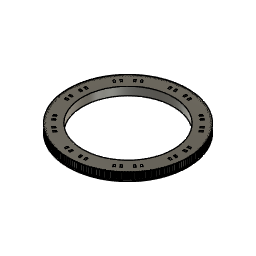
180 tooth pulley v3 (Autodesk Fusion 360 design; units mm, degrees)
Autodesk Fusion 360 part; units mm, degrees
(part 1 of 6)
sketch "Sketch1" plane through (0, 0, 0) normal (0, 0, 1) x (1, 0, 0)
  circle A0 centre (0, 0) radius 140.9967 construction
  circle A1 centre (0, 0) radius 143.2467 construction
  line L0 (0, 0) -> (143.2467, 0) construction
  line L1 (0, 0) -> (143.2249, 2.5) construction
  line L2 (143.2467, 0) -> (143.2467, 0.325)
  arc A2 (143.2467, 0.325) -> (142.786, 0.8235) centre (142.7467, 0.325) ccw
  arc A3 (140.9752, 2.4607) -> (142.786, 0.8235) centre (142.9432, 2.8173) ccw
  arc A4 (142.786, -0.8235) -> (140.9752, -2.4607) centre (142.9432, -2.8173) ccw
  arc A5 (142.786, -0.8235) -> (143.2467, -0.325) centre (142.7467, -0.325) ccw
  line L3 (143.2467, 0) -> (143.2467, -0.325)
  arc A6 (140.8035, 7.3792) -> (142.6703, 5.8061) centre (142.7578, 7.8042) ccw
  arc A7 (143.1481, 5.324) -> (142.6703, 5.8061) centre (142.6484, 5.3066) ccw
  line L4 (143.1595, 4.9992) -> (143.1481, 5.324)
  line L5 (143.1595, 4.9992) -> (143.1708, 4.6744)
  arc A8 (142.7278, 4.1602) -> (143.1708, 4.6744) centre (142.6711, 4.657) ccw
  arc A9 (142.7278, 4.1602) -> (140.9752, 2.4607) centre (142.9545, 2.1731) ccw
  arc A10 (140.4602, 12.2887) -> (142.3808, 10.7817) centre (142.3985, 12.7816) ccw
  arc A11 (142.8751, 10.3166) -> (142.3808, 10.7817) centre (142.3763, 10.2817) ccw
  line L6 (142.8978, 9.9924) -> (142.8751, 10.3166)
  line L7 (142.8978, 9.9924) -> (142.9205, 9.6682)
  arc A12 (142.4956, 9.1388) -> (142.9205, 9.6682) centre (142.4217, 9.6333) ccw
  arc A13 (142.4956, 9.1388) -> (140.8035, 7.3792) centre (142.7915, 7.1608) ccw
  arc A14 (139.9458, 17.1832) -> (141.9177, 15.7441) centre (141.8657, 17.7435) ccw
  arc A15 (142.428, 15.2966) -> (141.9177, 15.7441) centre (141.9308, 15.2443) ccw
  line L8 (142.462, 14.9734) -> (142.428, 15.2966)
  line L9 (142.462, 14.9734) -> (142.496, 14.6501)
  arc A16 (142.0899, 14.1063) -> (142.496, 14.6501) centre (141.9987, 14.5979) ccw
  arc A17 (142.0899, 14.1063) -> (140.4602, 12.2887) centre (142.4546, 12.1398) ccw
  arc A18 (139.2608, 22.0567) -> (141.2818, 20.6874) centre (141.16, 22.6837) ccw
  arc A19 (141.8074, 20.2579) -> (141.2818, 20.6874) centre (141.3123, 20.1883) ccw
  line L10 (141.8527, 19.9361) -> (141.8074, 20.2579)
  line L11 (141.8527, 19.9361) -> (141.8979, 19.6143)
  arc A20 (141.511, 19.0565) -> (141.8979, 19.6143) centre (141.4028, 19.5447) ccw
  arc A21 (141.511, 19.0565) -> (139.9458, 17.1832) centre (141.9442, 17.104) ccw
  arc A22 (138.4062, 26.9034) -> (140.4738, 25.6055) centre (140.2824, 27.5963) ccw
  arc A23 (141.014, 25.1946) -> (140.4738, 25.6055) centre (140.5216, 25.1078) ccw
  line L12 (141.0705, 24.8745) -> (141.014, 25.1946)
  line L13 (141.0705, 24.8745) -> (141.1269, 24.5545)
  arc A24 (140.7598, 23.9836) -> (141.1269, 24.5545) centre (140.6345, 24.4676) ccw
  arc A25 (140.7598, 23.9836) -> (139.2608, 22.0567) centre (141.2608, 22.0474) ccw
  arc A26 (137.383, 31.7174) -> (139.4946, 30.4923) centre (139.2338, 32.4753) ccw
  arc A27 (140.0489, 30.1006) -> (139.4946, 30.4923) centre (139.5598, 29.9966) ccw
  line L14 (140.1164, 29.7827) -> (140.0489, 30.1006)
  line L15 (140.1164, 29.7827) -> (140.184, 29.4648)
  arc A28 (139.837, 28.8814) -> (140.184, 29.4648) centre (139.6949, 29.3608) ccw
  arc A29 (139.837, 28.8814) -> (138.4062, 26.9034) centre (140.4053, 26.9639) ccw
  arc A30 (136.1924, 36.4926) -> (138.3455, 35.3421) centre (138.0156, 37.3147) ccw
  arc A31 (138.9131, 34.9699) -> (138.3455, 35.3421) centre (138.4279, 34.8489) ccw
  line L16 (138.9917, 34.6545) -> (138.9131, 34.9699)
  line L17 (138.9917, 34.6545) -> (139.0703, 34.3392)
  arc A32 (138.7439, 33.7441) -> (139.0703, 34.3392) centre (138.5852, 34.2182) ccw
  arc A33 (138.7439, 33.7441) -> (137.383, 31.7174) centre (139.3787, 31.8475) ccw
  arc A34 (134.8358, 41.2235) -> (137.0278, 40.1487) centre (136.6293, 42.1086) ccw
  arc A35 (137.608, 39.7966) -> (137.0278, 40.1487) centre (137.1274, 39.6587) ccw
  line L18 (137.6976, 39.4841) -> (137.608, 39.7966)
  line L19 (137.6976, 39.4841) -> (137.7872, 39.1717)
  arc A36 (137.4817, 38.5656) -> (137.7872, 39.1717) centre (137.3065, 39.0339) ccw
  arc A37 (137.4817, 38.5656) -> (136.1924, 36.4926) centre (138.1824, 36.6924) ccw
  arc A38 (133.315, 45.904) -> (135.5431, 44.9065) centre (135.0765, 46.8513) ccw
  arc A39 (136.1353, 44.5748) -> (135.5431, 44.9065) centre (135.6598, 44.4203) ccw
  line L20 (136.2357, 44.2657) -> (136.1353, 44.5748)
  line L21 (136.2357, 44.2657) -> (136.3362, 43.9566)
  arc A40 (136.052, 43.3402) -> (136.3362, 43.9566) centre (135.8606, 43.8021) ccw
  arc A41 (136.052, 43.3402) -> (134.8358, 41.2235) centre (136.8177, 41.4925) ccw
  arc A42 (131.6318, 50.5287) -> (133.8933, 49.6095) centre (133.3591, 51.5368) ccw
  arc A43 (134.4967, 49.2987) -> (133.8933, 49.6095) centre (134.0269, 49.1277) ccw
  line L22 (134.6079, 48.9933) -> (134.4967, 49.2987)
  line L23 (134.6079, 48.9933) -> (134.719, 48.6879)
  arc A44 (134.4566, 48.0619) -> (134.719, 48.6879) centre (134.2492, 48.5169) ccw
  arc A45 (134.4566, 48.0619) -> (133.315, 45.904) centre (135.2862, 46.2421) ccw
  arc A46 (129.7882, 55.0918) -> (132.0804, 54.2521) centre (131.4793, 56.1596) ccw
  arc A47 (132.6943, 53.9625) -> (132.0804, 54.2521) centre (132.2307, 53.7752) ccw
  line L24 (132.816, 53.6612) -> (132.6943, 53.9625)
  line L25 (132.816, 53.6612) -> (132.9378, 53.3598)
  arc A48 (132.6974, 52.7251) -> (132.9378, 53.3598) centre (132.4742, 53.1725) ccw
  arc A49 (132.6974, 52.7251) -> (131.6318, 50.5287) centre (133.59, 50.9353) ccw
  arc A50 (127.7864, 59.5878) -> (130.1066, 58.8286) centre (129.4392, 60.7139) ccw
  arc A51 (130.7302, 58.5606) -> (130.1066, 58.8286) centre (130.2734, 58.3572) ccw
  line L26 (130.8624, 58.2637) -> (130.7302, 58.5606)
  line L27 (130.8624, 58.2637) -> (130.9946, 57.9668)
  arc A52 (130.7764, 57.324) -> (130.9946, 57.9668) centre (130.5378, 57.7634) ccw
  arc A53 (130.7764, 57.324) -> (129.7882, 55.0918) centre (131.731, 55.5665) ccw
  arc A54 (125.629, 64.0112) -> (127.9742, 63.3334) centre (127.2415, 65.1943) ccw
  arc A55 (128.6068, 63.0873) -> (127.9742, 63.3334) centre (128.1574, 62.8682) ccw
  line L28 (128.7493, 62.7952) -> (128.6068, 63.0873)
  line L29 (128.7493, 62.7952) -> (128.8918, 62.5031)
  arc A56 (128.6962, 61.8532) -> (128.8918, 62.5031) centre (128.4424, 62.2839) ccw
  arc A57 (128.6962, 61.8532) -> (127.7864, 59.5878) centre (129.7115, 60.13) ccw
  arc A58 (123.3185, 68.3566) -> (125.686, 67.761) centre (124.8887, 69.5953) ccw
  arc A59 (126.3268, 67.5372) -> (125.686, 67.761) centre (125.8853, 67.3025) ccw
  line L30 (126.4793, 67.2503) -> (126.3268, 67.5372)
  line L31 (126.4793, 67.2503) -> (126.6319, 66.9633)
  arc A60 (126.4592, 66.3069) -> (126.6319, 66.9633) centre (126.1905, 66.7286) ccw
  arc A61 (126.4592, 66.3069) -> (125.629, 64.0112) centre (127.534, 64.6203) ccw
  arc A62 (120.8578, 72.6187) -> (123.2446, 72.1061) centre (122.3838, 73.9114) ccw
  arc A63 (123.8928, 71.9048) -> (123.2446, 72.1061) centre (123.4598, 71.6548) ccw
  line L32 (124.0553, 71.6234) -> (123.8928, 71.9048)
  line L33 (124.0553, 71.6234) -> (124.2178, 71.3419)
  arc A64 (124.068, 70.6799) -> (124.2178, 71.3419) centre (123.7848, 71.0919) ccw
  arc A65 (124.068, 70.6799) -> (123.3185, 68.3566) centre (125.2011, 69.0318) ccw
  arc A66 (118.2498, 76.7923) -> (120.653, 76.3634) centre (119.7298, 78.1375) ccw
  arc A67 (121.3079, 76.1848) -> (120.653, 76.3634) centre (120.8839, 75.9199) ccw
  line L34 (121.4801, 75.9092) -> (121.3079, 76.1848)
  line L35 (121.4801, 75.9092) -> (121.6523, 75.6336)
  arc A68 (121.5258, 74.9667) -> (121.6523, 75.6336) centre (121.2283, 75.3686) ccw
  arc A69 (121.5258, 74.9667) -> (120.8578, 72.6187) centre (122.7156, 73.3592) ccw
  arc A70 (115.4978, 80.8724) -> (117.9145, 80.5276) centre (116.9299, 82.2684) ccw
  arc A71 (118.5752, 80.372) -> (117.9145, 80.5276) centre (118.1607, 80.0924) ccw
  line L36 (118.7569, 80.1025) -> (118.5752, 80.372)
  line L37 (118.7569, 80.1025) -> (118.9387, 79.8331)
  arc A72 (118.8354, 79.1623) -> (118.9387, 79.8331) centre (118.5241, 79.5535) ccw
  arc A73 (118.8354, 79.1623) -> (118.2498, 76.7923) centre (120.0807, 77.5972) ccw
  arc A74 (112.605, 84.8539) -> (115.0323, 84.5937) centre (113.9875, 86.2991) ccw
  arc A75 (115.698, 84.4612) -> (115.0323, 84.5937) centre (115.2935, 84.1673) ccw
  line L38 (115.889, 84.1983) -> (115.698, 84.4612)
  line L39 (115.889, 84.1983) -> (116.0801, 83.9354)
  arc A76 (116.0003, 83.2613) -> (116.0801, 83.9354) centre (115.6756, 83.6415) ccw
  arc A77 (116.0003, 83.2613) -> (115.4978, 80.8724) centre (117.2994, 81.7407) ccw
  arc A78 (109.575, 88.7321) -> (112.01, 88.5567) centre (110.9063, 90.2247) ccw
  arc A79 (112.6799, 88.4476) -> (112.01, 88.5567) centre (112.2859, 88.1398) ccw
  line L40 (112.88, 88.1915) -> (112.6799, 88.4476)
  line L41 (112.88, 88.1915) -> (113.08, 87.9354)
  arc A80 (113.0239, 87.259) -> (113.08, 87.9354) centre (112.686, 87.6276) ccw
  arc A81 (113.0239, 87.259) -> (112.605, 84.8539) centre (114.3753, 85.7846) ccw
  arc A82 (106.4116, 92.5022) -> (108.8511, 92.4119) centre (107.6899, 94.0403) ccw
  arc A83 (109.5244, 92.3262) -> (108.8511, 92.4119) centre (109.1414, 92.0048) ccw
  line L42 (109.7334, 92.0772) -> (109.5244, 92.3262)
  line L43 (109.7334, 92.0772) -> (109.9423, 91.8283)
  arc A84 (109.9097, 91.1503) -> (109.9423, 91.8283) centre (109.5592, 91.5069) ccw
  arc A85 (109.9097, 91.1503) -> (109.575, 88.7321) centre (111.3118, 89.724) ccw
  arc A86 (103.1185, 96.1595) -> (105.5597, 96.1544) centre (104.3424, 97.7413) ccw
  arc A87 (106.2356, 96.0923) -> (105.5597, 96.1544) centre (105.864, 95.7577) ccw
  line L44 (106.4531, 95.8508) -> (106.2356, 96.0923)
  line L45 (106.4531, 95.8508) -> (106.6705, 95.6092)
  arc A88 (106.6617, 94.9306) -> (106.6705, 95.6092) centre (106.299, 95.2747) ccw
  arc A89 (106.6617, 94.9306) -> (106.4116, 92.5022) centre (108.1126, 93.554) ccw
  arc A90 (99.6997, 99.6997) -> (102.1396, 99.7798) centre (100.8677, 101.3233) ccw
  arc A91 (102.8173, 99.7413) -> (102.1396, 99.7798) centre (102.4576, 99.394) ccw
  line L46 (103.0431, 99.5075) -> (102.8173, 99.7413)
  line L47 (103.0431, 99.5075) -> (103.2688, 99.2737)
  arc A92 (103.2837, 98.5952) -> (103.2688, 99.2737) centre (102.9092, 98.9264) ccw
  arc A93 (103.2837, 98.5952) -> (103.1185, 96.1595) centre (104.7818, 97.2701) ccw
  arc A94 (96.1595, 103.1185) -> (98.5952, 103.2837) centre (97.2701, 104.7818) ccw
  arc A95 (99.2737, 103.2688) -> (98.5952, 103.2837) centre (98.9264, 102.9092) ccw
  line L48 (99.5075, 103.0431) -> (99.2737, 103.2688)
  line L49 (99.5075, 103.0431) -> (99.7413, 102.8173)
  arc A96 (99.7798, 102.1396) -> (99.7413, 102.8173) centre (99.394, 102.4576) ccw
  arc A97 (99.7798, 102.1396) -> (99.6997, 99.6997) centre (101.3233, 100.8677) ccw
  arc A98 (92.5022, 106.4116) -> (94.9306, 106.6617) centre (93.554, 108.1126) ccw
  arc A99 (95.6092, 106.6705) -> (94.9306, 106.6617) centre (95.2747, 106.299) ccw
  line L50 (95.8508, 106.4531) -> (95.6092, 106.6705)
  line L51 (95.8508, 106.4531) -> (96.0923, 106.2356)
  arc A100 (96.1544, 105.5597) -> (96.0923, 106.2356) centre (95.7577, 105.864) ccw
  arc A101 (96.1544, 105.5597) -> (96.1595, 103.1185) centre (97.7413, 104.3424) ccw
  arc A102 (88.7321, 109.575) -> (91.1503, 109.9097) centre (89.724, 111.3118) ccw
  arc A103 (91.8283, 109.9423) -> (91.1503, 109.9097) centre (91.5069, 109.5592) ccw
  line L52 (92.0772, 109.7334) -> (91.8283, 109.9423)
  line L53 (92.0772, 109.7334) -> (92.3262, 109.5244)
  arc A104 (92.4119, 108.8511) -> (92.3262, 109.5244) centre (92.0048, 109.1414) ccw
  arc A105 (92.4119, 108.8511) -> (92.5022, 106.4116) centre (94.0403, 107.6899) ccw
  arc A106 (84.8539, 112.605) -> (87.259, 113.0239) centre (85.7846, 114.3753) ccw
  arc A107 (87.9354, 113.08) -> (87.259, 113.0239) centre (87.6276, 112.686) ccw
  line L54 (88.1915, 112.88) -> (87.9354, 113.08)
  line L55 (88.1915, 112.88) -> (88.4476, 112.6799)
  arc A108 (88.5567, 112.01) -> (88.4476, 112.6799) centre (88.1398, 112.2859) ccw
  arc A109 (88.5567, 112.01) -> (88.7321, 109.575) centre (90.2247, 110.9063) ccw
  arc A110 (80.8724, 115.4978) -> (83.2613, 116.0003) centre (81.7407, 117.2994) ccw
  arc A111 (83.9354, 116.0801) -> (83.2613, 116.0003) centre (83.6415, 115.6756) ccw
  line L56 (84.1983, 115.889) -> (83.9354, 116.0801)
  line L57 (84.1983, 115.889) -> (84.4612, 115.698)
  arc A112 (84.5937, 115.0323) -> (84.4612, 115.698) centre (84.1673, 115.2935) ccw
  arc A113 (84.5937, 115.0323) -> (84.8539, 112.605) centre (86.2991, 113.9875) ccw
  arc A114 (76.7923, 118.2498) -> (79.1623, 118.8354) centre (77.5972, 120.0807) ccw
  arc A115 (79.8331, 118.9387) -> (79.1623, 118.8354) centre (79.5535, 118.5241) ccw
  line L58 (80.1025, 118.7569) -> (79.8331, 118.9387)
  line L59 (80.1025, 118.7569) -> (80.372, 118.5752)
  arc A116 (80.5276, 117.9145) -> (80.372, 118.5752) centre (80.0924, 118.1607) ccw
  arc A117 (80.5276, 117.9145) -> (80.8724, 115.4978) centre (82.2684, 116.9299) ccw
  arc A118 (72.6187, 120.8578) -> (74.9667, 121.5258) centre (73.3592, 122.7156) ccw
  arc A119 (75.6336, 121.6523) -> (74.9667, 121.5258) centre (75.3686, 121.2283) ccw
  line L60 (75.9092, 121.4801) -> (75.6336, 121.6523)
  line L61 (75.9092, 121.4801) -> (76.1848, 121.3079)
  arc A120 (76.3634, 120.653) -> (76.1848, 121.3079) centre (75.9199, 120.8839) ccw
  arc A121 (76.3634, 120.653) -> (76.7923, 118.2498) centre (78.1375, 119.7298) ccw
  arc A122 (68.3566, 123.3185) -> (70.6799, 124.068) centre (69.0318, 125.2011) ccw
  arc A123 (71.3419, 124.2178) -> (70.6799, 124.068) centre (71.0919, 123.7848) ccw
  line L62 (71.6234, 124.0553) -> (71.3419, 124.2178)
  line L63 (71.6234, 124.0553) -> (71.9048, 123.8928)
  arc A124 (72.1061, 123.2446) -> (71.9048, 123.8928) centre (71.6548, 123.4598) ccw
  arc A125 (72.1061, 123.2446) -> (72.6187, 120.8578) centre (73.9114, 122.3838) ccw
  arc A126 (64.0112, 125.629) -> (66.3069, 126.4592) centre (64.6203, 127.534) ccw
  arc A127 (66.9633, 126.6319) -> (66.3069, 126.4592) centre (66.7286, 126.1905) ccw
  line L64 (67.2503, 126.4793) -> (66.9633, 126.6319)
  line L65 (67.2503, 126.4793) -> (67.5372, 126.3268)
  arc A128 (67.761, 125.686) -> (67.5372, 126.3268) centre (67.3025, 125.8853) ccw
  arc A129 (67.761, 125.686) -> (68.3566, 123.3185) centre (69.5953, 124.8887) ccw
  arc A130 (59.5878, 127.7864) -> (61.8532, 128.6962) centre (60.13, 129.7115) ccw
  arc A131 (62.5031, 128.8918) -> (61.8532, 128.6962) centre (62.2839, 128.4424) ccw
  line L66 (62.7952, 128.7493) -> (62.5031, 128.8918)
  line L67 (62.7952, 128.7493) -> (63.0873, 128.6068)
  arc A132 (63.3334, 127.9742) -> (63.0873, 128.6068) centre (62.8682, 128.1574) ccw
  arc A133 (63.3334, 127.9742) -> (64.0112, 125.629) centre (65.1943, 127.2415) ccw
  arc A134 (55.0918, 129.7882) -> (57.324, 130.7764) centre (55.5665, 131.731) ccw
  arc A135 (57.9668, 130.9946) -> (57.324, 130.7764) centre (57.7634, 130.5378) ccw
  line L68 (58.2637, 130.8624) -> (57.9668, 130.9946)
  line L69 (58.2637, 130.8624) -> (58.5606, 130.7302)
  arc A136 (58.8286, 130.1066) -> (58.5606, 130.7302) centre (58.3572, 130.2734) ccw
  arc A137 (58.8286, 130.1066) -> (59.5878, 127.7864) centre (60.7139, 129.4392) ccw
  arc A138 (50.5287, 131.6318) -> (52.7251, 132.6974) centre (50.9353, 133.59) ccw
  arc A139 (53.3598, 132.9378) -> (52.7251, 132.6974) centre (53.1725, 132.4742) ccw
  line L70 (53.6612, 132.816) -> (53.3598, 132.9378)
  line L71 (53.6612, 132.816) -> (53.9625, 132.6943)
  arc A140 (54.2521, 132.0804) -> (53.9625, 132.6943) centre (53.7752, 132.2307) ccw
  arc A141 (54.2521, 132.0804) -> (55.0918, 129.7882) centre (56.1596, 131.4793) ccw
  arc A142 (45.904, 133.315) -> (48.0619, 134.4566) centre (46.2421, 135.2862) ccw
  arc A143 (48.6879, 134.719) -> (48.0619, 134.4566) centre (48.5169, 134.2492) ccw
  line L72 (48.9933, 134.6079) -> (48.6879, 134.719)
  line L73 (48.9933, 134.6079) -> (49.2987, 134.4967)
  arc A144 (49.6095, 133.8933) -> (49.2987, 134.4967) centre (49.1277, 134.0269) ccw
  arc A145 (49.6095, 133.8933) -> (50.5287, 131.6318) centre (51.5368, 133.3591) ccw
  arc A146 (41.2235, 134.8358) -> (43.3402, 136.052) centre (41.4925, 136.8177) ccw
  arc A147 (43.9566, 136.3362) -> (43.3402, 136.052) centre (43.8021, 135.8606) ccw
  line L74 (44.2657, 136.2357) -> (43.9566, 136.3362)
  line L75 (44.2657, 136.2357) -> (44.5748, 136.1353)
  arc A148 (44.9065, 135.5431) -> (44.5748, 136.1353) centre (44.4203, 135.6598) ccw
  arc A149 (44.9065, 135.5431) -> (45.904, 133.315) centre (46.8513, 135.0765) ccw
  arc A150 (36.4926, 136.1924) -> (38.5656, 137.4817) centre (36.6924, 138.1824) ccw
  arc A151 (39.1717, 137.7872) -> (38.5656, 137.4817) centre (39.0339, 137.3065) ccw
  line L76 (39.4841, 137.6976) -> (39.1717, 137.7872)
  line L77 (39.4841, 137.6976) -> (39.7966, 137.608)
  arc A152 (40.1487, 137.0278) -> (39.7966, 137.608) centre (39.6587, 137.1274) ccw
  arc A153 (40.1487, 137.0278) -> (41.2235, 134.8358) centre (42.1086, 136.6293) ccw
  arc A154 (31.7174, 137.383) -> (33.7441, 138.7439) centre (31.8475, 139.3787) ccw
  arc A155 (34.3392, 139.0703) -> (33.7441, 138.7439) centre (34.2182, 138.5852) ccw
  line L78 (34.6545, 138.9917) -> (34.3392, 139.0703)
  line L79 (34.6545, 138.9917) -> (34.9699, 138.9131)
  arc A156 (35.3421, 138.3455) -> (34.9699, 138.9131) centre (34.8489, 138.4279) ccw
  arc A157 (35.3421, 138.3455) -> (36.4926, 136.1924) centre (37.3147, 138.0156) ccw
  arc A158 (26.9034, 138.4062) -> (28.8814, 139.837) centre (26.9639, 140.4053) ccw
  arc A159 (29.4648, 140.184) -> (28.8814, 139.837) centre (29.3608, 139.6949) ccw
  line L80 (29.7827, 140.1164) -> (29.4648, 140.184)
  line L81 (29.7827, 140.1164) -> (30.1006, 140.0489)
  arc A160 (30.4923, 139.4946) -> (30.1006, 140.0489) centre (29.9966, 139.5598) ccw
  arc A161 (30.4923, 139.4946) -> (31.7174, 137.383) centre (32.4753, 139.2338) ccw
  arc A162 (22.0567, 139.2608) -> (23.9836, 140.7598) centre (22.0474, 141.2608) ccw
  arc A163 (24.5545, 141.1269) -> (23.9836, 140.7598) centre (24.4676, 140.6345) ccw
  line L82 (24.8745, 141.0705) -> (24.5545, 141.1269)
  line L83 (24.8745, 141.0705) -> (25.1946, 141.014)
  arc A164 (25.6055, 140.4738) -> (25.1946, 141.014) centre (25.1078, 140.5216) ccw
  arc A165 (25.6055, 140.4738) -> (26.9034, 138.4062) centre (27.5963, 140.2824) ccw
  arc A166 (17.1832, 139.9458) -> (19.0565, 141.511) centre (17.104, 141.9442) ccw
  arc A167 (19.6143, 141.8979) -> (19.0565, 141.511) centre (19.5447, 141.4028) ccw
  line L84 (19.9361, 141.8527) -> (19.6143, 141.8979)
  line L85 (19.9361, 141.8527) -> (20.2579, 141.8074)
  arc A168 (20.6874, 141.2818) -> (20.2579, 141.8074) centre (20.1883, 141.3123) ccw
  arc A169 (20.6874, 141.2818) -> (22.0567, 139.2608) centre (22.6837, 141.16) ccw
  arc A170 (12.2887, 140.4602) -> (14.1063, 142.0899) centre (12.1398, 142.4546) ccw
  arc A171 (14.6501, 142.496) -> (14.1063, 142.0899) centre (14.5979, 141.9987) ccw
  line L86 (14.9734, 142.462) -> (14.6501, 142.496)
  line L87 (14.9734, 142.462) -> (15.2966, 142.428)
  arc A172 (15.7441, 141.9177) -> (15.2966, 142.428) centre (15.2443, 141.9308) ccw
  arc A173 (15.7441, 141.9177) -> (17.1832, 139.9458) centre (17.7435, 141.8657) ccw
  arc A174 (7.3792, 140.8035) -> (9.1388, 142.4956) centre (7.1608, 142.7915) ccw
  arc A175 (9.6682, 142.9205) -> (9.1388, 142.4956) centre (9.6333, 142.4217) ccw
  line L88 (9.9924, 142.8978) -> (9.6682, 142.9205)
  line L89 (9.9924, 142.8978) -> (10.3166, 142.8751)
  arc A176 (10.7817, 142.3808) -> (10.3166, 142.8751) centre (10.2817, 142.3763) ccw
  arc A177 (10.7817, 142.3808) -> (12.2887, 140.4602) centre (12.7816, 142.3985) ccw
  arc A178 (2.4607, 140.9752) -> (4.1602, 142.7278) centre (2.1731, 142.9545) ccw
  arc A179 (4.6744, 143.1708) -> (4.1602, 142.7278) centre (4.657, 142.6711) ccw
  line L90 (4.9992, 143.1595) -> (4.6744, 143.1708)
  line L91 (4.9992, 143.1595) -> (5.324, 143.1481)
  arc A180 (5.8061, 142.6703) -> (5.324, 143.1481) centre (5.3066, 142.6484) ccw
  arc A181 (5.8061, 142.6703) -> (7.3792, 140.8035) centre (7.8042, 142.7578) ccw
  arc A182 (-2.4607, 140.9752) -> (-0.8235, 142.786) centre (-2.8173, 142.9432) ccw
  arc A183 (-0.325, 143.2467) -> (-0.8235, 142.786) centre (-0.325, 142.7467) ccw
  line L92 (0, 143.2467) -> (-0.325, 143.2467)
  line L93 (0, 143.2467) -> (0.325, 143.2467)
  arc A184 (0.8235, 142.786) -> (0.325, 143.2467) centre (0.325, 142.7467) ccw
  arc A185 (0.8235, 142.786) -> (2.4607, 140.9752) centre (2.8173, 142.9432) ccw
  arc A186 (-7.3792, 140.8035) -> (-5.8061, 142.6703) centre (-7.8042, 142.7578) ccw
  arc A187 (-5.324, 143.1481) -> (-5.8061, 142.6703) centre (-5.3066, 142.6484) ccw
  line L94 (-4.9992, 143.1595) -> (-5.324, 143.1481)
  line L95 (-4.9992, 143.1595) -> (-4.6744, 143.1708)
  arc A188 (-4.1602, 142.7278) -> (-4.6744, 143.1708) centre (-4.657, 142.6711) ccw
  arc A189 (-4.1602, 142.7278) -> (-2.4607, 140.9752) centre (-2.1731, 142.9545) ccw
  arc A190 (-12.2887, 140.4602) -> (-10.7817, 142.3808) centre (-12.7816, 142.3985) ccw
  arc A191 (-10.3166, 142.8751) -> (-10.7817, 142.3808) centre (-10.2817, 142.3763) ccw
  line L96 (-9.9924, 142.8978) -> (-10.3166, 142.8751)
  line L97 (-9.9924, 142.8978) -> (-9.6682, 142.9205)
  arc A192 (-9.1388, 142.4956) -> (-9.6682, 142.9205) centre (-9.6333, 142.4217) ccw
  arc A193 (-9.1388, 142.4956) -> (-7.3792, 140.8035) centre (-7.1608, 142.7915) ccw
  arc A194 (-17.1832, 139.9458) -> (-15.7441, 141.9177) centre (-17.7435, 141.8657) ccw
  arc A195 (-15.2966, 142.428) -> (-15.7441, 141.9177) centre (-15.2443, 141.9308) ccw
  line L98 (-14.9734, 142.462) -> (-15.2966, 142.428)
  line L99 (-14.9734, 142.462) -> (-14.6501, 142.496)
  arc A196 (-14.1063, 142.0899) -> (-14.6501, 142.496) centre (-14.5979, 141.9987) ccw
  arc A197 (-14.1063, 142.0899) -> (-12.2887, 140.4602) centre (-12.1398, 142.4546) ccw
  arc A198 (-22.0567, 139.2608) -> (-20.6874, 141.2818) centre (-22.6837, 141.16) ccw
  arc A199 (-20.2579, 141.8074) -> (-20.6874, 141.2818) centre (-20.1883, 141.3123) ccw
  line L100 (-19.9361, 141.8527) -> (-20.2579, 141.8074)
  line L101 (-19.9361, 141.8527) -> (-19.6143, 141.8979)
  arc A200 (-19.0565, 141.511) -> (-19.6143, 141.8979) centre (-19.5447, 141.4028) ccw
  arc A201 (-19.0565, 141.511) -> (-17.1832, 139.9458) centre (-17.104, 141.9442) ccw
  arc A202 (-26.9034, 138.4062) -> (-25.6055, 140.4738) centre (-27.5963, 140.2824) ccw
  arc A203 (-25.1946, 141.014) -> (-25.6055, 140.4738) centre (-25.1078, 140.5216) ccw
  line L102 (-24.8745, 141.0705) -> (-25.1946, 141.014)
  line L103 (-24.8745, 141.0705) -> (-24.5545, 141.1269)
  arc A204 (-23.9836, 140.7598) -> (-24.5545, 141.1269) centre (-24.4676, 140.6345) ccw
  arc A205 (-23.9836, 140.7598) -> (-22.0567, 139.2608) centre (-22.0474, 141.2608) ccw
  arc A206 (-31.7174, 137.383) -> (-30.4923, 139.4946) centre (-32.4753, 139.2338) ccw
  arc A207 (-30.1006, 140.0489) -> (-30.4923, 139.4946) centre (-29.9966, 139.5598) ccw
  line L104 (-29.7827, 140.1164) -> (-30.1006, 140.0489)
  line L105 (-29.7827, 140.1164) -> (-29.4648, 140.184)
  arc A208 (-28.8814, 139.837) -> (-29.4648, 140.184) centre (-29.3608, 139.6949) ccw
  arc A209 (-28.8814, 139.837) -> (-26.9034, 138.4062) centre (-26.9639, 140.4053) ccw
  arc A210 (-36.4926, 136.1924) -> (-35.3421, 138.3455) centre (-37.3147, 138.0156) ccw
  arc A211 (-34.9699, 138.9131) -> (-35.3421, 138.3455) centre (-34.8489, 138.4279) ccw
  line L106 (-34.6545, 138.9917) -> (-34.9699, 138.9131)
  line L107 (-34.6545, 138.9917) -> (-34.3392, 139.0703)
  arc A212 (-33.7441, 138.7439) -> (-34.3392, 139.0703) centre (-34.2182, 138.5852) ccw
  arc A213 (-33.7441, 138.7439) -> (-31.7174, 137.383) centre (-31.8475, 139.3787) ccw
  arc A214 (-41.2235, 134.8358) -> (-40.1487, 137.0278) centre (-42.1086, 136.6293) ccw
  arc A215 (-39.7966, 137.608) -> (-40.1487, 137.0278) centre (-39.6587, 137.1274) ccw
  line L108 (-39.4841, 137.6976) -> (-39.7966, 137.608)
  line L109 (-39.4841, 137.6976) -> (-39.1717, 137.7872)
  arc A216 (-38.5656, 137.4817) -> (-39.1717, 137.7872) centre (-39.0339, 137.3065) ccw
  arc A217 (-38.5656, 137.4817) -> (-36.4926, 136.1924) centre (-36.6924, 138.1824) ccw
  arc A218 (-45.904, 133.315) -> (-44.9065, 135.5431) centre (-46.8513, 135.0765) ccw
  arc A219 (-44.5748, 136.1353) -> (-44.9065, 135.5431) centre (-44.4203, 135.6598) ccw
  line L110 (-44.2657, 136.2357) -> (-44.5748, 136.1353)
  line L111 (-44.2657, 136.2357) -> (-43.9566, 136.3362)
  arc A220 (-43.3402, 136.052) -> (-43.9566, 136.3362) centre (-43.8021, 135.8606) ccw
  arc A221 (-43.3402, 136.052) -> (-41.2235, 134.8358) centre (-41.4925, 136.8177) ccw
  arc A222 (-50.5287, 131.6318) -> (-49.6095, 133.8933) centre (-51.5368, 133.3591) ccw
  arc A223 (-49.2987, 134.4967) -> (-49.6095, 133.8933) centre (-49.1277, 134.0269) ccw
  line L112 (-48.9933, 134.6079) -> (-49.2987, 134.4967)
  line L113 (-48.9933, 134.6079) -> (-48.6879, 134.719)
  arc A224 (-48.0619, 134.4566) -> (-48.6879, 134.719) centre (-48.5169, 134.2492) ccw
  arc A225 (-48.0619, 134.4566) -> (-45.904, 133.315) centre (-46.2421, 135.2862) ccw
  arc A226 (-55.0918, 129.7882) -> (-54.2521, 132.0804) centre (-56.1596, 131.4793) ccw
  arc A227 (-53.9625, 132.6943) -> (-54.2521, 132.0804) centre (-53.7752, 132.2307) ccw
  line L114 (-53.6612, 132.816) -> (-53.9625, 132.6943)
  line L115 (-53.6612, 132.816) -> (-53.3598, 132.9378)
  arc A228 (-52.7251, 132.6974) -> (-53.3598, 132.9378) centre (-53.1725, 132.4742) ccw
  arc A229 (-52.7251, 132.6974) -> (-50.5287, 131.6318) centre (-50.9353, 133.59) ccw
  arc A230 (-59.5878, 127.7864) -> (-58.8286, 130.1066) centre (-60.7139, 129.4392) ccw
  arc A231 (-58.5606, 130.7302) -> (-58.8286, 130.1066) centre (-58.3572, 130.2734) ccw
  line L116 (-58.2637, 130.8624) -> (-58.5606, 130.7302)
  line L117 (-58.2637, 130.8624) -> (-57.9668, 130.9946)
  arc A232 (-57.324, 130.7764) -> (-57.9668, 130.9946) centre (-57.7634, 130.5378) ccw
  arc A233 (-57.324, 130.7764) -> (-55.0918, 129.7882) centre (-55.5665, 131.731) ccw
  arc A234 (-64.0112, 125.629) -> (-63.3334, 127.9742) centre (-65.1943, 127.2415) ccw
  arc A235 (-63.0873, 128.6068) -> (-63.3334, 127.9742) centre (-62.8682, 128.1574) ccw
  line L118 (-62.7952, 128.7493) -> (-63.0873, 128.6068)
  line L119 (-62.7952, 128.7493) -> (-62.5031, 128.8918)
  arc A236 (-61.8532, 128.6962) -> (-62.5031, 128.8918) centre (-62.2839, 128.4424) ccw
  arc A237 (-61.8532, 128.6962) -> (-59.5878, 127.7864) centre (-60.13, 129.7115) ccw
  arc A238 (-68.3566, 123.3185) -> (-67.761, 125.686) centre (-69.5953, 124.8887) ccw
  arc A239 (-67.5372, 126.3268) -> (-67.761, 125.686) centre (-67.3025, 125.8853) ccw
  line L120 (-67.2503, 126.4793) -> (-67.5372, 126.3268)
  line L121 (-67.2503, 126.4793) -> (-66.9633, 126.6319)
  arc A240 (-66.3069, 126.4592) -> (-66.9633, 126.6319) centre (-66.7286, 126.1905) ccw
  arc A241 (-66.3069, 126.4592) -> (-64.0112, 125.629) centre (-64.6203, 127.534) ccw
  arc A242 (-72.6187, 120.8578) -> (-72.1061, 123.2446) centre (-73.9114, 122.3838) ccw
  arc A243 (-71.9048, 123.8928) -> (-72.1061, 123.2446) centre (-71.6548, 123.4598) ccw
  line L122 (-71.6234, 124.0553) -> (-71.9048, 123.8928)
  line L123 (-71.6234, 124.0553) -> (-71.3419, 124.2178)
  arc A244 (-70.6799, 124.068) -> (-71.3419, 124.2178) centre (-71.0919, 123.7848) ccw
  arc A245 (-70.6799, 124.068) -> (-68.3566, 123.3185) centre (-69.0318, 125.2011) ccw
  arc A246 (-76.7923, 118.2498) -> (-76.3634, 120.653) centre (-78.1375, 119.7298) ccw
  arc A247 (-76.1848, 121.3079) -> (-76.3634, 120.653) centre (-75.9199, 120.8839) ccw
  line L124 (-75.9092, 121.4801) -> (-76.1848, 121.3079)
  line L125 (-75.9092, 121.4801) -> (-75.6336, 121.6523)
  arc A248 (-74.9667, 121.5258) -> (-75.6336, 121.6523) centre (-75.3686, 121.2283) ccw
  arc A249 (-74.9667, 121.5258) -> (-72.6187, 120.8578) centre (-73.3592, 122.7156) ccw
  arc A250 (-80.8724, 115.4978) -> (-80.5276, 117.9145) centre (-82.2684, 116.9299) ccw
  arc A251 (-80.372, 118.5752) -> (-80.5276, 117.9145) centre (-80.0924, 118.1607) ccw
  line L126 (-80.1025, 118.7569) -> (-80.372, 118.5752)
  line L127 (-80.1025, 118.7569) -> (-79.8331, 118.9387)
  arc A252 (-79.1623, 118.8354) -> (-79.8331, 118.9387) centre (-79.5535, 118.5241) ccw
  arc A253 (-79.1623, 118.8354) -> (-76.7923, 118.2498) centre (-77.5972, 120.0807) ccw
  arc A254 (-84.8539, 112.605) -> (-84.5937, 115.0323) centre (-86.2991, 113.9875) ccw
  arc A255 (-84.4612, 115.698) -> (-84.5937, 115.0323) centre (-84.1673, 115.2935) ccw
  line L128 (-84.1983, 115.889) -> (-84.4612, 115.698)
  line L129 (-84.1983, 115.889) -> (-83.9354, 116.0801)
  arc A256 (-83.2613, 116.0003) -> (-83.9354, 116.0801) centre (-83.6415, 115.6756) ccw
  arc A257 (-83.2613, 116.0003) -> (-80.8724, 115.4978) centre (-81.7407, 117.2994) ccw
  arc A258 (-88.7321, 109.575) -> (-88.5567, 112.01) centre (-90.2247, 110.9063) ccw
  arc A259 (-88.4476, 112.6799) -> (-88.5567, 112.01) centre (-88.1398, 112.2859) ccw
  line L130 (-88.1915, 112.88) -> (-88.4476, 112.6799)
  line L131 (-88.1915, 112.88) -> (-87.9354, 113.08)
  arc A260 (-87.259, 113.0239) -> (-87.9354, 113.08) centre (-87.6276, 112.686) ccw
  arc A261 (-87.259, 113.0239) -> (-84.8539, 112.605) centre (-85.7846, 114.3753) ccw
  arc A262 (-92.5022, 106.4116) -> (-92.4119, 108.8511) centre (-94.0403, 107.6899) ccw
  arc A263 (-92.3262, 109.5244) -> (-92.4119, 108.8511) centre (-92.0048, 109.1414) ccw
  line L132 (-92.0772, 109.7334) -> (-92.3262, 109.5244)
  line L133 (-92.0772, 109.7334) -> (-91.8283, 109.9423)
  arc A264 (-91.1503, 109.9097) -> (-91.8283, 109.9423) centre (-91.5069, 109.5592) ccw
  arc A265 (-91.1503, 109.9097) -> (-88.7321, 109.575) centre (-89.724, 111.3118) ccw
  arc A266 (-96.1595, 103.1185) -> (-96.1544, 105.5597) centre (-97.7413, 104.3424) ccw
  arc A267 (-96.0923, 106.2356) -> (-96.1544, 105.5597) centre (-95.7577, 105.864) ccw
  line L134 (-95.8508, 106.4531) -> (-96.0923, 106.2356)
  line L135 (-95.8508, 106.4531) -> (-95.6092, 106.6705)
  arc A268 (-94.9306, 106.6617) -> (-95.6092, 106.6705) centre (-95.2747, 106.299) ccw
  arc A269 (-94.9306, 106.6617) -> (-92.5022, 106.4116) centre (-93.554, 108.1126) ccw
  arc A270 (-99.6997, 99.6997) -> (-99.7798, 102.1396) centre (-101.3233, 100.8677) ccw
  arc A271 (-99.7413, 102.8173) -> (-99.7798, 102.1396) centre (-99.394, 102.4576) ccw
  line L136 (-99.5075, 103.0431) -> (-99.7413, 102.8173)
  line L137 (-99.5075, 103.0431) -> (-99.2737, 103.2688)
  arc A272 (-98.5952, 103.2837) -> (-99.2737, 103.2688) centre (-98.9264, 102.9092) ccw
  arc A273 (-98.5952, 103.2837) -> (-96.1595, 103.1185) centre (-97.2701, 104.7818) ccw
  arc A274 (-103.1185, 96.1595) -> (-103.2837, 98.5952) centre (-104.7818, 97.2701) ccw
  arc A275 (-103.2688, 99.2737) -> (-103.2837, 98.5952) centre (-102.9092, 98.9264) ccw
  line L138 (-103.0431, 99.5075) -> (-103.2688, 99.2737)
  line L139 (-103.0431, 99.5075) -> (-102.8173, 99.7413)
  arc A276 (-102.1396, 99.7798) -> (-102.8173, 99.7413) centre (-102.4576, 99.394) ccw
  arc A277 (-102.1396, 99.7798) -> (-99.6997, 99.6997) centre (-100.8677, 101.3233) ccw
  arc A278 (-106.4116, 92.5022) -> (-106.6617, 94.9306) centre (-108.1126, 93.554) ccw
  arc A279 (-106.6705, 95.6092) -> (-106.6617, 94.9306) centre (-106.299, 95.2747) ccw
  line L140 (-106.4531, 95.8508) -> (-106.6705, 95.6092)
  line L141 (-106.4531, 95.8508) -> (-106.2356, 96.0923)
  arc A280 (-105.5597, 96.1544) -> (-106.2356, 96.0923) centre (-105.864, 95.7577) ccw
  arc A281 (-105.5597, 96.1544) -> (-103.1185, 96.1595) centre (-104.3424, 97.7413) ccw
  arc A282 (-109.575, 88.7321) -> (-109.9097, 91.1503) centre (-111.3118, 89.724) ccw
  arc A283 (-109.9423, 91.8283) -> (-109.9097, 91.1503) centre (-109.5592, 91.5069) ccw
  line L142 (-109.7334, 92.0772) -> (-109.9423, 91.8283)
  line L143 (-109.7334, 92.0772) -> (-109.5244, 92.3262)
  arc A284 (-108.8511, 92.4119) -> (-109.5244, 92.3262) centre (-109.1414, 92.0048) ccw
  arc A285 (-108.8511, 92.4119) -> (-106.4116, 92.5022) centre (-107.6899, 94.0403) ccw
  arc A286 (-112.605, 84.8539) -> (-113.0239, 87.259) centre (-114.3753, 85.7846) ccw
  arc A287 (-113.08, 87.9354) -> (-113.0239, 87.259) centre (-112.686, 87.6276) ccw
  line L144 (-112.88, 88.1915) -> (-113.08, 87.9354)
  line L145 (-112.88, 88.1915) -> (-112.6799, 88.4476)
  arc A288 (-112.01, 88.5567) -> (-112.6799, 88.4476) centre (-112.2859, 88.1398) ccw
  arc A289 (-112.01, 88.5567) -> (-109.575, 88.7321) centre (-110.9063, 90.2247) ccw
  arc A290 (-115.4978, 80.8724) -> (-116.0003, 83.2613) centre (-117.2994, 81.7407) ccw
  arc A291 (-116.0801, 83.9354) -> (-116.0003, 83.2613) centre (-115.6756, 83.6415) ccw
  line L146 (-115.889, 84.1983) -> (-116.0801, 83.9354)
  line L147 (-115.889, 84.1983) -> (-115.698, 84.4612)
  arc A292 (-115.0323, 84.5937) -> (-115.698, 84.4612) centre (-115.2935, 84.1673) ccw
  arc A293 (-115.0323, 84.5937) -> (-112.605, 84.8539) centre (-113.9875, 86.2991) ccw
  arc A294 (-118.2498, 76.7923) -> (-118.8354, 79.1623) centre (-120.0807, 77.5972) ccw
  arc A295 (-118.9387, 79.8331) -> (-118.8354, 79.1623) centre (-118.5241, 79.5535) ccw
  line L148 (-118.7569, 80.1025) -> (-118.9387, 79.8331)
  line L149 (-118.7569, 80.1025) -> (-118.5752, 80.372)
  arc A296 (-117.9145, 80.5276) -> (-118.5752, 80.372) centre (-118.1607, 80.0924) ccw
  arc A297 (-117.9145, 80.5276) -> (-115.4978, 80.8724) centre (-116.9299, 82.2684) ccw
  arc A298 (-120.8578, 72.6187) -> (-121.5258, 74.9667) centre (-122.7156, 73.3592) ccw
  arc A299 (-121.6523, 75.6336) -> (-121.5258, 74.9667) centre (-121.2283, 75.3686) ccw
  line L150 (-121.4801, 75.9092) -> (-121.6523, 75.6336)
  line L151 (-121.4801, 75.9092) -> (-121.3079, 76.1848)
  arc A300 (-120.653, 76.3634) -> (-121.3079, 76.1848) centre (-120.8839, 75.9199) ccw
  arc A301 (-120.653, 76.3634) -> (-118.2498, 76.7923) centre (-119.7298, 78.1375) ccw
  arc A302 (-123.3185, 68.3566) -> (-124.068, 70.6799) centre (-125.2011, 69.0318) ccw
  arc A303 (-124.2178, 71.3419) -> (-124.068, 70.6799) centre (-123.7848, 71.0919) ccw
  line L152 (-124.0553, 71.6234) -> (-124.2178, 71.3419)
  line L153 (-124.0553, 71.6234) -> (-123.8928, 71.9048)
  arc A304 (-123.2446, 72.1061) -> (-123.8928, 71.9048) centre (-123.4598, 71.6548) ccw
  arc A305 (-123.2446, 72.1061) -> (-120.8578, 72.6187) centre (-122.3838, 73.9114) ccw
  arc A306 (-125.629, 64.0112) -> (-126.4592, 66.3069) centre (-127.534, 64.6203) ccw
  arc A307 (-126.6319, 66.9633) -> (-126.4592, 66.3069) centre (-126.1905, 66.7286) ccw
  line L154 (-126.4793, 67.2503) -> (-126.6319, 66.9633)
  line L155 (-126.4793, 67.2503) -> (-126.3268, 67.5372)
  arc A308 (-125.686, 67.761) -> (-126.3268, 67.5372) centre (-125.8853, 67.3025) ccw
  arc A309 (-125.686, 67.761) -> (-123.3185, 68.3566) centre (-124.8887, 69.5953) ccw
  arc A310 (-127.7864, 59.5878) -> (-128.6962, 61.8532) centre (-129.7115, 60.13) ccw
  arc A311 (-128.8918, 62.5031) -> (-128.6962, 61.8532) centre (-128.4424, 62.2839) ccw
  line L156 (-128.7493, 62.7952) -> (-128.8918, 62.5031)
  line L157 (-128.7493, 62.7952) -> (-128.6068, 63.0873)
  arc A312 (-127.9742, 63.3334) -> (-128.6068, 63.0873) centre (-128.1574, 62.8682) ccw
  arc A313 (-127.9742, 63.3334) -> (-125.629, 64.0112) centre (-127.2415, 65.1943) ccw
  arc A314 (-129.7882, 55.0918) -> (-130.7764, 57.324) centre (-131.731, 55.5665) ccw
  arc A315 (-130.9946, 57.9668) -> (-130.7764, 57.324) centre (-130.5378, 57.7634) ccw
  line L158 (-130.8624, 58.2637) -> (-130.9946, 57.9668)
  line L159 (-130.8624, 58.2637) -> (-130.7302, 58.5606)
  arc A316 (-130.1066, 58.8286) -> (-130.7302, 58.5606) centre (-130.2734, 58.3572) ccw
  arc A317 (-130.1066, 58.8286) -> (-127.7864, 59.5878) centre (-129.4392, 60.7139) ccw
  arc A318 (-131.6318, 50.5287) -> (-132.6974, 52.7251) centre (-133.59, 50.9353) ccw
  arc A319 (-132.9378, 53.3598) -> (-132.6974, 52.7251) centre (-132.4742, 53.1725) ccw
  line L160 (-132.816, 53.6612) -> (-132.9378, 53.3598)
  line L161 (-132.816, 53.6612) -> (-132.6943, 53.9625)
  arc A320 (-132.0804, 54.2521) -> (-132.6943, 53.9625) centre (-132.2307, 53.7752) ccw
  arc A321 (-132.0804, 54.2521) -> (-129.7882, 55.0918) centre (-131.4793, 56.1596) ccw
  arc A322 (-133.315, 45.904) -> (-134.4566, 48.0619) centre (-135.2862, 46.2421) ccw
  arc A323 (-134.719, 48.6879) -> (-134.4566, 48.0619) centre (-134.2492, 48.5169) ccw
  line L162 (-134.6079, 48.9933) -> (-134.719, 48.6879)
  line L163 (-134.6079, 48.9933) -> (-134.4967, 49.2987)
  arc A324 (-133.8933, 49.6095) -> (-134.4967, 49.2987) centre (-134.0269, 49.1277) ccw
  arc A325 (-133.8933, 49.6095) -> (-131.6318, 50.5287) centre (-133.3591, 51.5368) ccw
  arc A326 (-134.8358, 41.2235) -> (-136.052, 43.3402) centre (-136.8177, 41.4925) ccw
  arc A327 (-136.3362, 43.9566) -> (-136.052, 43.3402) centre (-135.8606, 43.8021) ccw
  line L164 (-136.2357, 44.2657) -> (-136.3362, 43.9566)
  line L165 (-136.2357, 44.2657) -> (-136.1353, 44.5748)
  arc A328 (-135.5431, 44.9065) -> (-136.1353, 44.5748) centre (-135.6598, 44.4203) ccw
  arc A329 (-135.5431, 44.9065) -> (-133.315, 45.904) centre (-135.0765, 46.8513) ccw
  arc A330 (-136.1924, 36.4926) -> (-137.4817, 38.5656) centre (-138.1824, 36.6924) ccw
  arc A331 (-137.7872, 39.1717) -> (-137.4817, 38.5656) centre (-137.3065, 39.0339) ccw
  line L166 (-137.6976, 39.4841) -> (-137.7872, 39.1717)
  line L167 (-137.6976, 39.4841) -> (-137.608, 39.7966)
  arc A332 (-137.0278, 40.1487) -> (-137.608, 39.7966) centre (-137.1274, 39.6587) ccw
  arc A333 (-137.0278, 40.1487) -> (-134.8358, 41.2235) centre (-136.6293, 42.1086) ccw
  arc A334 (-137.383, 31.7174) -> (-138.7439, 33.7441) centre (-139.3787, 31.8475) ccw
  arc A335 (-139.0703, 34.3392) -> (-138.7439, 33.7441) centre (-138.5852, 34.2182) ccw
  line L168 (-138.9917, 34.6545) -> (-139.0703, 34.3392)
  line L169 (-138.9917, 34.6545) -> (-138.9131, 34.9699)
  arc A336 (-138.3455, 35.3421) -> (-138.9131, 34.9699) centre (-138.4279, 34.8489) ccw
  arc A337 (-138.3455, 35.3421) -> (-136.1924, 36.4926) centre (-138.0156, 37.3147) ccw
  arc A338 (-138.4062, 26.9034) -> (-139.837, 28.8814) centre (-140.4053, 26.9639) ccw
  arc A339 (-140.184, 29.4648) -> (-139.837, 28.8814) centre (-139.6949, 29.3608) ccw
  line L170 (-140.1164, 29.7827) -> (-140.184, 29.4648)
  line L171 (-140.1164, 29.7827) -> (-140.0489, 30.1006)
  arc A340 (-139.4946, 30.4923) -> (-140.0489, 30.1006) centre (-139.5598, 29.9966) ccw
  arc A341 (-139.4946, 30.4923) -> (-137.383, 31.7174) centre (-139.2338, 32.4753) ccw
  arc A342 (-139.2608, 22.0567) -> (-140.7598, 23.9836) centre (-141.2608, 22.0474) ccw
  arc A343 (-141.1269, 24.5545) -> (-140.7598, 23.9836) centre (-140.6345, 24.4676) ccw
  line L172 (-141.0705, 24.8745) -> (-141.1269, 24.5545)
  line L173 (-141.0705, 24.8745) -> (-141.014, 25.1946)
  arc A344 (-140.4738, 25.6055) -> (-141.014, 25.1946) centre (-140.5216, 25.1078) ccw
  arc A345 (-140.4738, 25.6055) -> (-138.4062, 26.9034) centre (-140.2824, 27.5963) ccw
  arc A346 (-139.9458, 17.1832) -> (-141.511, 19.0565) centre (-141.9442, 17.104) ccw
  arc A347 (-141.8979, 19.6143) -> (-141.511, 19.0565) centre (-141.4028, 19.5447) ccw
  line L174 (-141.8527, 19.9361) -> (-141.8979, 19.6143)
  line L175 (-141.8527, 19.9361) -> (-141.8074, 20.2579)
  arc A348 (-141.2818, 20.6874) -> (-141.8074, 20.2579) centre (-141.3123, 20.1883) ccw
  arc A349 (-141.2818, 20.6874) -> (-139.2608, 22.0567) centre (-141.16, 22.6837) ccw
  arc A350 (-140.4602, 12.2887) -> (-142.0899, 14.1063) centre (-142.4546, 12.1398) ccw
  arc A351 (-142.496, 14.6501) -> (-142.0899, 14.1063) centre (-141.9987, 14.5979) ccw
  line L176 (-142.462, 14.9734) -> (-142.496, 14.6501)
  line L177 (-142.462, 14.9734) -> (-142.428, 15.2966)
  arc A352 (-141.9177, 15.7441) -> (-142.428, 15.2966) centre (-141.9308, 15.2443) ccw
  arc A353 (-141.9177, 15.7441) -> (-139.9458, 17.1832) centre (-141.8657, 17.7435) ccw
  arc A354 (-140.8035, 7.3792) -> (-142.4956, 9.1388) centre (-142.7915, 7.1608) ccw
  arc A355 (-142.9205, 9.6682) -> (-142.4956, 9.1388) centre (-142.4217, 9.6333) ccw
  line L178 (-142.8978, 9.9924) -> (-142.9205, 9.6682)
  line L179 (-142.8978, 9.9924) -> (-142.8751, 10.3166)
  arc A356 (-142.3808, 10.7817) -> (-142.8751, 10.3166) centre (-142.3763, 10.2817) ccw
  arc A357 (-142.3808, 10.7817) -> (-140.4602, 12.2887) centre (-142.3985, 12.7816) ccw
  arc A358 (-140.9752, 2.4607) -> (-142.7278, 4.1602) centre (-142.9545, 2.1731) ccw
  arc A359 (-143.1708, 4.6744) -> (-142.7278, 4.1602) centre (-142.6711, 4.657) ccw
  line L180 (-143.1595, 4.9992) -> (-143.1708, 4.6744)
  line L181 (-143.1595, 4.9992) -> (-143.1481, 5.324)
  arc A360 (-142.6703, 5.8061) -> (-143.1481, 5.324) centre (-142.6484, 5.3066) ccw
  arc A361 (-142.6703, 5.8061) -> (-140.8035, 7.3792) centre (-142.7578, 7.8042) ccw
  arc A362 (-140.9752, -2.4607) -> (-142.786, -0.8235) centre (-142.9432, -2.8173) ccw
  arc A363 (-143.2467, -0.325) -> (-142.786, -0.8235) centre (-142.7467, -0.325) ccw
  line L182 (-143.2467, 0) -> (-143.2467, -0.325)
  line L183 (-143.2467, 0) -> (-143.2467, 0.325)
  arc A364 (-142.786, 0.8235) -> (-143.2467, 0.325) centre (-142.7467, 0.325) ccw
  arc A365 (-142.786, 0.8235) -> (-140.9752, 2.4607) centre (-142.9432, 2.8173) ccw
  arc A366 (-140.8035, -7.3792) -> (-142.6703, -5.8061) centre (-142.7578, -7.8042) ccw
  arc A367 (-143.1481, -5.324) -> (-142.6703, -5.8061) centre (-142.6484, -5.3066) ccw
  line L184 (-143.1595, -4.9992) -> (-143.1481, -5.324)
  line L185 (-143.1595, -4.9992) -> (-143.1708, -4.6744)
  arc A368 (-142.7278, -4.1602) -> (-143.1708, -4.6744) centre (-142.6711, -4.657) ccw
  arc A369 (-142.7278, -4.1602) -> (-140.9752, -2.4607) centre (-142.9545, -2.1731) ccw
  arc A370 (-140.4602, -12.2887) -> (-142.3808, -10.7817) centre (-142.3985, -12.7816) ccw
  arc A371 (-142.8751, -10.3166) -> (-142.3808, -10.7817) centre (-142.3763, -10.2817) ccw
  line L186 (-142.8978, -9.9924) -> (-142.8751, -10.3166)
  line L187 (-142.8978, -9.9924) -> (-142.9205, -9.6682)
  arc A372 (-142.4956, -9.1388) -> (-142.9205, -9.6682) centre (-142.4217, -9.6333) ccw
  arc A373 (-142.4956, -9.1388) -> (-140.8035, -7.3792) centre (-142.7915, -7.1608) ccw
  arc A374 (-139.9458, -17.1832) -> (-141.9177, -15.7441) centre (-141.8657, -17.7435) ccw
  arc A375 (-142.428, -15.2966) -> (-141.9177, -15.7441) centre (-141.9308, -15.2443) ccw
  line L188 (-142.462, -14.9734) -> (-142.428, -15.2966)
  line L189 (-142.462, -14.9734) -> (-142.496, -14.6501)
  arc A376 (-142.0899, -14.1063) -> (-142.496, -14.6501) centre (-141.9987, -14.5979) ccw
  arc A377 (-142.0899, -14.1063) -> (-140.4602, -12.2887) centre (-142.4546, -12.1398) ccw
  arc A378 (-139.2608, -22.0567) -> (-141.2818, -20.6874) centre (-141.16, -22.6837) ccw
  arc A379 (-141.8074, -20.2579) -> (-141.2818, -20.6874) centre (-141.3123, -20.1883) ccw
  line L190 (-141.8527, -19.9361) -> (-141.8074, -20.2579)
  line L191 (-141.8527, -19.9361) -> (-141.8979, -19.6143)
  arc A380 (-141.511, -19.0565) -> (-141.8979, -19.6143) centre (-141.4028, -19.5447) ccw
  arc A381 (-141.511, -19.0565) -> (-139.9458, -17.1832) centre (-141.9442, -17.104) ccw
  arc A382 (-138.4062, -26.9034) -> (-140.4738, -25.6055) centre (-140.2824, -27.5963) ccw
  arc A383 (-141.014, -25.1946) -> (-140.4738, -25.6055) centre (-140.5216, -25.1078) ccw
  line L192 (-141.0705, -24.8745) -> (-141.014, -25.1946)
  line L193 (-141.0705, -24.8745) -> (-141.1269, -24.5545)
  arc A384 (-140.7598, -23.9836) -> (-141.1269, -24.5545) centre (-140.6345, -24.4676) ccw
  arc A385 (-140.7598, -23.9836) -> (-139.2608, -22.0567) centre (-141.2608, -22.0474) ccw
  arc A386 (-137.383, -31.7174) -> (-139.4946, -30.4923) centre (-139.2338, -32.4753) ccw
  arc A387 (-140.0489, -30.1006) -> (-139.4946, -30.4923) centre (-139.5598, -29.9966) ccw
  line L194 (-140.1164, -29.7827) -> (-140.0489, -30.1006)
  line L195 (-140.1164, -29.7827) -> (-140.184, -29.4648)
  arc A388 (-139.837, -28.8814) -> (-140.184, -29.4648) centre (-139.6949, -29.3608) ccw
  arc A389 (-139.837, -28.8814) -> (-138.4062, -26.9034) centre (-140.4053, -26.9639) ccw
  arc A390 (-136.1924, -36.4926) -> (-138.3455, -35.3421) centre (-138.0156, -37.3147) ccw
  arc A391 (-138.9131, -34.9699) -> (-138.3455, -35.3421) centre (-138.4279, -34.8489) ccw
  line L196 (-138.9917, -34.6545) -> (-138.9131, -34.9699)
  line L197 (-138.9917, -34.6545) -> (-139.0703, -34.3392)
  arc A392 (-138.7439, -33.7441) -> (-139.0703, -34.3392) centre (-138.5852, -34.2182) ccw
  arc A393 (-138.7439, -33.7441) -> (-137.383, -31.7174) centre (-139.3787, -31.8475) ccw
  arc A394 (-134.8358, -41.2235) -> (-137.0278, -40.1487) centre (-136.6293, -42.1086) ccw
  arc A395 (-137.608, -39.7966) -> (-137.0278, -40.1487) centre (-137.1274, -39.6587) ccw
  line L198 (-137.6976, -39.4841) -> (-137.608, -39.7966)
  line L199 (-137.6976, -39.4841) -> (-137.7872, -39.1717)
  arc A396 (-137.4817, -38.5656) -> (-137.7872, -39.1717) centre (-137.3065, -39.0339) ccw
  arc A397 (-137.4817, -38.5656) -> (-136.1924, -36.4926) centre (-138.1824, -36.6924) ccw
  arc A398 (-133.315, -45.904) -> (-135.5431, -44.9065) centre (-135.0765, -46.8513) ccw
  arc A399 (-136.1353, -44.5748) -> (-135.5431, -44.9065) centre (-135.6598, -44.4203) ccw
  line L200 (-136.2357, -44.2657) -> (-136.1353, -44.5748)
  line L201 (-136.2357, -44.2657) -> (-136.3362, -43.9566)
  arc A400 (-136.052, -43.3402) -> (-136.3362, -43.9566) centre (-135.8606, -43.8021) ccw
  arc A401 (-136.052, -43.3402) -> (-134.8358, -41.2235) centre (-136.8177, -41.4925) ccw
  arc A402 (-131.6318, -50.5287) -> (-133.8933, -49.6095) centre (-133.3591, -51.5368) ccw
  arc A403 (-134.4967, -49.2987) -> (-133.8933, -49.6095) centre (-134.0269, -49.1277) ccw
  line L202 (-134.6079, -48.9933) -> (-134.4967, -49.2987)
  line L203 (-134.6079, -48.9933) -> (-134.719, -48.6879)
  arc A404 (-134.4566, -48.0619) -> (-134.719, -48.6879) centre (-134.2492, -48.5169) ccw
  arc A405 (-134.4566, -48.0619) -> (-133.315, -45.904) centre (-135.2862, -46.2421) ccw
  arc A406 (-129.7882, -55.0918) -> (-132.0804, -54.2521) centre (-131.4793, -56.1596) ccw
  arc A407 (-132.6943, -53.9625) -> (-132.0804, -54.2521) centre (-132.2307, -53.7752) ccw
  line L204 (-132.816, -53.6612) -> (-132.6943, -53.9625)
  line L205 (-132.816, -53.6612) -> (-132.9378, -53.3598)
  arc A408 (-132.6974, -52.7251) -> (-132.9378, -53.3598) centre (-132.4742, -53.1725) ccw
  arc A409 (-132.6974, -52.7251) -> (-131.6318, -50.5287) centre (-133.59, -50.9353) ccw
  arc A410 (-127.7864, -59.5878) -> (-130.1066, -58.8286) centre (-129.4392, -60.7139) ccw
  arc A411 (-130.7302, -58.5606) -> (-130.1066, -58.8286) centre (-130.2734, -58.3572) ccw
  line L206 (-130.8624, -58.2637) -> (-130.7302, -58.5606)
  line L207 (-130.8624, -58.2637) -> (-130.9946, -57.9668)
  arc A412 (-130.7764, -57.324) -> (-130.9946, -57.9668) centre (-130.5378, -57.7634) ccw
  arc A413 (-130.7764, -57.324) -> (-129.7882, -55.0918) centre (-131.731, -55.5665) ccw
  arc A414 (-125.629, -64.0112) -> (-127.9742, -63.3334) centre (-127.2415, -65.1943) ccw
  arc A415 (-128.6068, -63.0873) -> (-127.9742, -63.3334) centre (-128.1574, -62.8682) ccw
  line L208 (-128.7493, -62.7952) -> (-128.6068, -63.0873)
  line L209 (-128.7493, -62.7952) -> (-128.8918, -62.5031)
  arc A416 (-128.6962, -61.8532) -> (-128.8918, -62.5031) centre (-128.4424, -62.2839) ccw
  arc A417 (-128.6962, -61.8532) -> (-127.7864, -59.5878) centre (-129.7115, -60.13) ccw
  arc A418 (-123.3185, -68.3566) -> (-125.686, -67.761) centre (-124.8887, -69.5953) ccw
  arc A419 (-126.3268, -67.5372) -> (-125.686, -67.761) centre (-125.8853, -67.3025) ccw
  line L210 (-126.4793, -67.2503) -> (-126.3268, -67.5372)
  line L211 (-126.4793, -67.2503) -> (-126.6319, -66.9633)
  arc A420 (-126.4592, -66.3069) -> (-126.6319, -66.9633) centre (-126.1905, -66.7286) ccw
  arc A421 (-126.4592, -66.3069) -> (-125.629, -64.0112) centre (-127.534, -64.6203) ccw
  arc A422 (-120.8578, -72.6187) -> (-123.2446, -72.1061) centre (-122.3838, -73.9114) ccw
  arc A423 (-123.8928, -71.9048) -> (-123.2446, -72.1061) centre (-123.4598, -71.6548) ccw
  line L212 (-124.0553, -71.6234) -> (-123.8928, -71.9048)
  line L213 (-124.0553, -71.6234) -> (-124.2178, -71.3419)
  arc A424 (-124.068, -70.6799) -> (-124.2178, -71.3419) centre (-123.7848, -71.0919) ccw
  arc A425 (-124.068, -70.6799) -> (-123.3185, -68.3566) centre (-125.2011, -69.0318) ccw
  arc A426 (-118.2498, -76.7923) -> (-120.653, -76.3634) centre (-119.7298, -78.1375) ccw
  arc A427 (-121.3079, -76.1848) -> (-120.653, -76.3634) centre (-120.8839, -75.9199) ccw
  line L214 (-121.4801, -75.9092) -> (-121.3079, -76.1848)
  line L215 (-121.4801, -75.9092) -> (-121.6523, -75.6336)
  arc A428 (-121.5258, -74.9667) -> (-121.6523, -75.6336) centre (-121.2283, -75.3686) ccw
  arc A429 (-121.5258, -74.9667) -> (-120.8578, -72.6187) centre (-122.7156, -73.3592) ccw
  arc A430 (-115.4978, -80.8724) -> (-117.9145, -80.5276) centre (-116.9299, -82.2684) ccw
  arc A431 (-118.5752, -80.372) -> (-117.9145, -80.5276) centre (-118.1607, -80.0924) ccw
  line L216 (-118.7569, -80.1025) -> (-118.5752, -80.372)
  line L217 (-118.7569, -80.1025) -> (-118.9387, -79.8331)
  arc A432 (-118.8354, -79.1623) -> (-118.9387, -79.8331) centre (-118.5241, -79.5535) ccw
  arc A433 (-118.8354, -79.1623) -> (-118.2498, -76.7923) centre (-120.0807, -77.5972) ccw
  arc A434 (-112.605, -84.8539) -> (-115.0323, -84.5937) centre (-113.9875, -86.2991) ccw
  arc A435 (-115.698, -84.4612) -> (-115.0323, -84.5937) centre (-115.2935, -84.1673) ccw
  line L218 (-115.889, -84.1983) -> (-115.698, -84.4612)
  line L219 (-115.889, -84.1983) -> (-116.0801, -83.9354)
  arc A436 (-116.0003, -83.2613) -> (-116.0801, -83.9354) centre (-115.6756, -83.6415) ccw